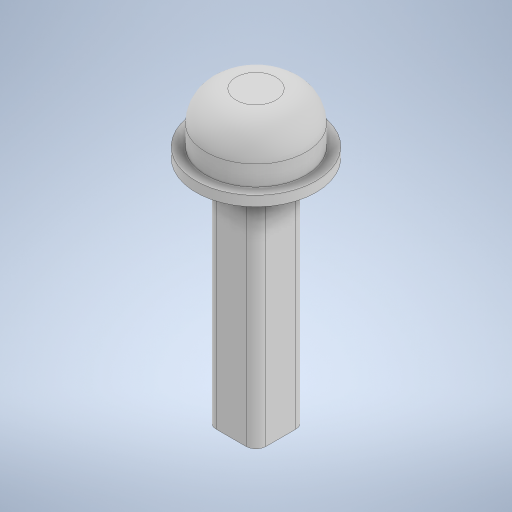
# Autodesk Inventor part: EvoTest_body
Saved by Autodesk Inventor 2023.2 (Build 272271000, 271)
## iProperties
Created: 2022-12-05
Part Number: EvoTest_body
Material: Generico
Document SubType Name: Modeling
Designer: Silvio Marano
Density: 1 g/cm^3
Appearance: Default
Engineer: Silvio Marano
Author: Silvio Marano
Title: EVOTest
Autodesk Inventor part; units mm, degrees
ref_plane "YZ Plane" through (0, 0, 0) normal (1, 0, 0) x (0, 1, 0)
ref_plane "XZ Plane" through (0, 0, 0) normal (0, 1, 0) x (-1, 0, 0)
ref_plane "XY Plane" through (0, 0, 0) normal (0, 0, 1) x (1, 0, 0)
sketch "MainSketch" plane through (0, 0, 0) normal (0, 1, 0) x (-1, 0, 0)
  line L0 (31, -50) -> (-31, -50)
  line L1 (-31, -50) -> (-31, 50)
  line L2 (-31, 50) -> (31, 50)
  line L3 (31, 50) -> (31, -50)
  line L4 (31, -49.4494) -> (-31, 50.5506) construction
  line L5 (-31, -50) -> (31, 50) construction
  line L6 (31, 50) -> (-31, 50)
  line L7 (-31, 50) -> (-31, 21.5)
  line L8 (-31, 21.5) -> (31, 21.5)
  line L9 (31, 21.5) -> (31, 50)
  line L10 (-31, -50) -> (16, -50)
  line L11 (16, -50) -> (16, 21.5)
  line L12 (16, 21.5) -> (-31, 21.5)
  line L13 (-31, 21.5) -> (-31, -50)
  line L14 (31, 21.5) -> (16, 21.5)
  line L15 (16, 21.5) -> (16, -50)
  line L16 (16, -50) -> (31, -50)
  line L17 (31, -50) -> (31, 21.5)
  line L18 (-31, 21.5) -> (-31, 35.75)
  line L19 (-31, 21.5) -> (-31, 35.75)
  arc A0 (0, 50) -> (-31, 21.5) centre (0.8091, 18.0102) ccw
  line L20 (29.5, 48.5) -> (-29.5, 48.5)
  line L21 (-29.5, 48.5) -> (-29.5, -48.5)
  line L22 (-29.5, -48.5) -> (29.5, -48.5)
  line L23 (29.5, -48.5) -> (29.5, 48.5)
  line L24 (29.5, 48.5) -> (-29.5, -48.5) construction
  line L25 (-29.5, 48.5) -> (29.5, -48.5) construction
  line L26 (-29.5, -48.5) -> (16, -48.5)
  line L27 (16, -48.5) -> (16, 2.2597)
  line L28 (16, 2.2597) -> (-29.5, 2.2597)
  line L29 (-29.5, 2.2597) -> (-29.5, -48.5)
  line L30 (16, -48.5) -> (29.5, -48.5)
  line L31 (29.5, -48.5) -> (29.5, 11.5)
  line L32 (29.5, 11.5) -> (16, 11.5)
  line L33 (16, 11.5) -> (16, -48.5)
  line L34 (29.5, 21.5) -> (16, 21.5)
  line L35 (16, 21.5) -> (16, 11.5)
  line L36 (16, 11.5) -> (29.5, 11.5)
  line L37 (29.5, 11.5) -> (29.5, 21.5)
  line L38 (29.5, 21.5) -> (29.5, 11.5)
  line L39 (29.5, 16.5) -> (16, 16.5)
  line L40 (22.75, 16.5) -> (22.75, 11.5)
  line L41 (22.75, 16.5) -> (22.75, 21.5)
  circle A1 centre (22.75, 16.5) radius 4
  arc A2 (0, 48.5) -> (-29.5, 21.5) centre (0.9166, 17.8828) ccw
  line L42 (-20.0675, 15.4609) -> (-7.0675, 15.4609)
  line L43 (-7.0675, 15.4609) -> (-7.0675, -23.5689)
  line L44 (-7.0675, -23.5689) -> (-20.0675, -23.5689)
  line L45 (-20.0675, -23.5689) -> (-20.0675, 15.4609)
  line L46 (22.75, 11.5) -> (22.75, -28.5)
  line L47 (22.75, 11.5) -> (62.75, 11.5) construction
  line L48 (20.2505, -33.5) -> (20.2505, -28.5)
  line L49 (22.75, -28.5) -> (25.2505, -28.5)
  line L50 (20.2505, -28.5) -> (25.2505, -28.5)
  line L51 (25.2505, -28.5) -> (25.2505, -33.5)
  line L52 (25.2505, -33.5) -> (20.2505, -33.5)
  line L53 (20.2505, -33.5) -> (20.2505, -28.5)
  line L54 (25.2505, -28.5) -> (20.2505, -33.5)
  line L55 (20.2505, -28.5) -> (25.2505, -33.5)
  circle A3 centre (22.7505, -31) radius 5
  line L56 (-7.0675, 15.4609) -> (-20.0675, 15.4609)
  line L57 (-20.0675, 15.4609) -> (-20.0675, 10.4609)
  line L58 (-20.0675, 10.4609) -> (-7.0675, 10.4609)
  line L59 (-7.0675, 10.4609) -> (-7.0675, 15.4609)
  line L60 (-7.0675, -23.5689) -> (-20.0675, -23.5689)
  line L61 (-20.0675, -23.5689) -> (-20.0675, -18.5689)
  line L62 (-20.0675, -18.5689) -> (-7.0675, -18.5689)
  line L63 (-7.0675, -18.5689) -> (-7.0675, -23.5689)
  line L64 (-29.5, -48.5) -> (-16.5, -48.5)
  line L65 (-16.5, -48.5) -> (-8.5, -48.5)
  line L66 (-8.5, -48.5) -> (-8.5, -42.5)
  line L67 (-8.5, -42.5) -> (-16.5, -42.5)
  line L68 (-16.5, -42.5) -> (-16.5, -48.5)
  line L69 (-8.5, -42.5) -> (-4.5, -42.5)
  line L70 (-8.5, -42.5) -> (-4.5, -42.5) construction
  line L71 (-4.5, -42.5) -> (-3.5, -42.5)
  line L72 (-3.5, -42.5) -> (-3.5, -40.5)
  line L73 (-3.5, -40.5) -> (-4.5, -40.5)
  line L74 (-4.5, -40.5) -> (-4.5, -42.5)
  line L75 (-4.5, -42.5) -> (-3.5, -42.5)
  line L76 (-3.5, -42.5) -> (-3.5, -44.5)
  line L77 (-3.5, -44.5) -> (-4.5, -44.5)
  line L78 (-4.5, -44.5) -> (-4.5, -42.5)
  line L79 (-8.5, -42.5) -> (-8.5, -10.5)
  line L80 (-8.5, -10.5) -> (-10.5, -10.5)
  line L81 (-10.5, -10.5) -> (-10.5, -9.5)
  line L82 (-10.5, -9.5) -> (-8.5, -9.5)
  line L83 (-8.5, -9.5) -> (-8.5, -10.5)
  line L84 (-8.5, -42.5) -> (-8.5, -37.5)
  line L85 (-8.5, -37.5) -> (-9.5, -37.5)
  line L86 (-9.5, -37.5) -> (-9.5, -39.5)
  line L87 (-9.5, -39.5) -> (-8.5, -39.5)
  line L88 (-8.5, -39.5) -> (-8.5, -37.5)
  point P0 (0, 0)
  dimension "d0" = 62
  dimension "d1" = 100
  dimension "d2" = 62
  dimension "d3" = 28.5
  dimension "d4" = 47
  dimension "d5" = 32
  dimension "d6" = 59
  dimension "d7" = 97
  dimension "d8" = 60
  dimension "d9" = 8
  dimension "d10" = 39.0299
  dimension "d11" = 13
  dimension "d12" = 40
  dimension "d13" = 90
  dimension "d14" = 5
  dimension "d15" = 5
  dimension "d16" = 10
  dimension "d17" = 5
  dimension "d18" = 5
  dimension "d19" = 13
  dimension "d20" = 8
  dimension "d21" = 6
  dimension "d22" = 4
  dimension "d23" = 0
  dimension "d24" = 1
  dimension "d25" = 2
  dimension "d26" = 2
  dimension "d27" = 32
  dimension "d28" = 2
  dimension "d29" = 1
  dimension "d30" = 5
  dimension "d31" = 1
  dimension "d32" = 2
  constraints: 178 end point, 32 parallel, 21 perpendicular, 19 horizontal, 12 midpoint, 12 point on line, 4 centre point, 4 point on circle, 2 equal length, 2 vertical, 1 coincident, 1 collinear
  measures "d0" distance of L2.start L2.end
  measures "d1" distance of L3.end L2.end
  measures "d2" distance of L8.end L7.end
  measures "d3" distance of L7.end L6.end
  measures "d4" distance of L12.end L11.end
  measures "d5" radius of A0
  measures "d6" distance of L22.end L21.end
  measures "d7" distance of L21.end L20.end
  measures "d8" distance of L31.end L30.end
  measures "d9" diameter of A1
  measures "d10" distance of L44.end L42.start
  measures "d11" distance of L43.end L44.end
  measures "d12" distance of L40.end L46.end
  measures "d13" angle of L46 L47
  measures "d14" distance of L51.end L48.start
  measures "d15" distance of L49.end L51.end
  measures "d16" diameter of A3
  measures "d17" distance of L57.end L56.end
  measures "d18" distance of L60.end L61.end
  measures "d19" distance of L21.end L64.end
  measures "d20" distance of L67.end L66.end
  measures "d21" distance of L66.end L65.end
  measures "d22" distance of L66.end L69.end
  measures "d23" distance between parallel lines of L69 L70
  measures "d24" distance of L73.end L72.end
  measures "d25" distance of L72.end L71.end
  measures "d26" distance of L75.end L76.end
  measures "d27" distance of L66.end L79.end
  measures "d28" distance of L79.end L80.end
  measures "d29" distance of L80.end L81.end
  measures "d30" distance of L66.end L84.end
  measures "d31" distance of L87.end L86.end
  measures "d32" distance of L86.end L85.end
extrude "MainExtrusion" add sketch "MainSketch" along normal blind 6 contours L49 L54 L55 L50 | A3 | L51 L55 L54 | L55 L54 L48 | L52 L54 L55
sketch "ButtonBlockerSketch" plane through (-22.7505, 0, -31) normal (0, -1, 0) x (1, 0, 0)
  circle A0 centre (0, 0) radius 6
  point P0 (22.7505, 31)
  dimension "d35" = 12
  constraints: 1 centre point
  measures "d35" diameter of A0
extrude "ButtonBlockerExtrusion" add sketch "ButtonBlockerSketch" against normal blind 1
fillet "MainConnection" radius 3 1 edges at (-17.7505, 6, -31)
sketch "ClickerProtusionSketch" plane through (-22.7505, 0, -31) normal (0, -1, 0) x (1, 0, 0)
  line L0 (2.5, 2.5) -> (-2.5, 2.5)
  line L1 (-2.5, 2.5) -> (-2.5, -2.5)
  line L2 (-2.5, -2.5) -> (2.5, -2.5)
  line L3 (2.5, -2.5) -> (2.5, 2.5)
  line L4 (2.5, 2.5) -> (-2.5, -2.5) construction
  line L5 (-2.5, 2.5) -> (2.5, -2.5) construction
  point P0 (22.7505, 31)
  point P1 (0, 0)
  dimension "d39" = 5
  dimension "d40" = 5
  constraints: 12 end point, 2 midpoint, 2 parallel, 1 horizontal, 1 perpendicular
  measures "d39" distance of L2.end L1.end
  measures "d40" distance of L1.end L0.end
extrude "ClickerProtusionExtrusion" add sketch "ClickerProtusionSketch" along normal blind 23
fillet "ClickerProtusionConnection" radius 1 4 edges at (-20.2505, -11.5, -33.5) (-20.2505, -11.5, -28.5) (-25.2505, -11.5, -33.5) (-25.2505, -11.5, -28.5)
